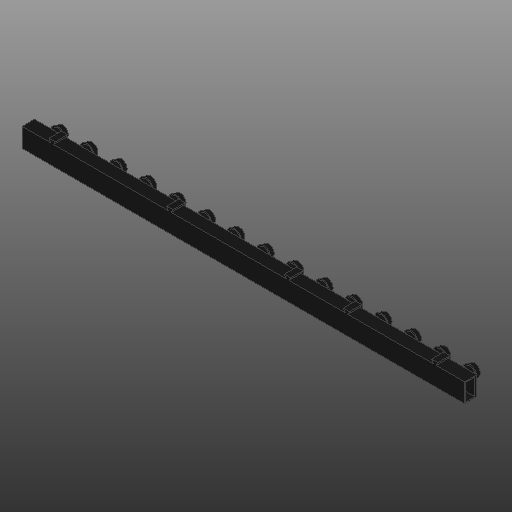
# Autodesk Inventor part: Manifold0
Saved by Autodesk Inventor 2020 (Build 240168000, 168)
## iProperties
Created: 2019-12-01
Part Number: Manifold0
Material: PLA Plastic (Black)
Document SubType Name: Modeling
Designer: Isaac Newcomb
Density: 1.06 g/cm^3
Appearance: 3D Printed - Black
Mass: 3.4119 g
Surface Area: 108.618 cm^2
Volume: 3.21878 cm^3
Project: Ice Keys
d33: 12.200 mm
d34: 2.533 mm
d35: 1.147 mm
d36: 1.300 mm
d37: 2.533 mm
d38: 1.147 mm
d39: 1.300 mm
d40: 2.533 mm
d41: 1.147 mm
d42: 1.300 mm
d43: 2.533 mm
d44: 1.147 mm
d45: 1.300 mm
d46: 2.533 mm
d47: 1.147 mm
d48: 1.300 mm
d53: 2.533 mm
d54: 1.147 mm
d55: 1.300 mm
d56: 2.533 mm
d57: 1.147 mm
d58: 1.300 mm
d61: 3.200 mm
d62: 1.600 mm
d63: 1.500 mm
d64: 3.200 mm
d65: 1.600 mm
d66: 1.500 mm
d67: 3.200 mm
d68: 1.600 mm
d69: 1.500 mm
d70: 3.200 mm
d71: 1.600 mm
d72: 1.500 mm
d73: 3.200 mm
d74: 1.600 mm
d75: 1.500 mm
d77: 0.400 mm
Author: Isaac Newcomb
Autodesk Inventor part; units mm, degrees
ref_plane "XZ Plane" through (0, 0, 0) normal (0, 1, 0) x (-1, 0, 0)
ref_plane "XY Plane" through (0, 0, 0) normal (0, 0, 1) x (1, 0, 0)
sketch "Box Sketch" plane through (0, 0, 0) normal (1, 0, 0) x (0, 1, 0)
  line L0 (0, 0) -> (7.7625, 0)
  line L1 (7.7625, 0) -> (7.7625, 5)
  line L2 (7.7625, 5) -> (0, 5)
  line L3 (0, 5) -> (0, 0)
  line L4 (0.4, 0.8) -> (7.3625, 0.8)
  line L5 (7.3625, 0.8) -> (7.3625, 4.6)
  line L6 (7.3625, 4.6) -> (0.4, 4.6)
  line L7 (0.4, 4.6) -> (0.4, 0.8)
  dimension "d0" = 0.8
  dimension "boxWallThick" = 0.4
  dimension "d2" = 0.4
  dimension "d3" = 0.4
  dimension "boxHeight" = 7.7625
  dimension "boxWidth" = 5
  constraints: 16 end point, 4 parallel, 2 horizontal, 2 perpendicular
  measures "d0" distance between parallel lines of L0 L4
  measures "boxWallThick" distance between parallel lines of L1 L5
  measures "d2" distance between parallel lines of L3 L7
  measures "d3" distance between parallel lines of L2 L6
  measures "boxHeight" distance of L0.start L0.end
  measures "boxWidth" distance of L2.end L0.start
extrude "Box" add sketch "Box Sketch" along normal blind 12.4
ref_plane "Fitting Plane" through (6.2, 0, 0) normal (1, 0, 0) x (0, 1, 0)
sketch "Fitting Sketch" plane through (6.2, 0, 0) normal (1, 0, 0) x (0, 1, 0)
  line L0 (3.8813, 0) -> (3.8813, -5.25) construction
  line L1 (5.4625, 0) -> (5.4625, -5.25)
  line L2 (5.4625, -5.25) -> (6.2625, -5.25)
  line L3 (6.2625, -5.25) -> (6.7625, -3.25)
  line L4 (6.7625, -3.25) -> (6.2625, -3.25)
  line L5 (6.2625, -3.25) -> (6.7625, -1.25)
  line L6 (6.7625, -1.25) -> (6.2625, -1.25)
  line L7 (6.2625, -1.25) -> (6.2625, 0)
  line L8 (6.2625, 0) -> (5.4625, 0)
  point P0 (0, 0)
  dimension "d10" = 2
  dimension "d11" = 0.5
  dimension "d12" = 1.25
  dimension "d13" = 0.8
  dimension "d14" = 2.3813
  dimension "d15" = 3.8813
  constraints: 18 end point, 5 point on line, 4 parallel, 3 perpendicular, 2 vertical
  measures "d10" distance between parallel lines of L6 L4
  measures "d11" distance of L3.end L4.end
  measures "d12" distance of L6.end L7.end
  measures "d13" distance of L1.end L2.end
  measures "d14" distance between parallel lines of L7 L0
  measures "d15" distance from line of point (0, 0) L0
revolve "Fitting" add sketch "Fitting Sketch" angle 360 about axis through (6.2, 3.8813, 0) along (0, 0, -1)
sketch "Fitting Entrance Sketch" plane through (6.2, 3.8813, 0) normal (0, 0, -1) x (-1, 0, 0)
  circle A0 centre (0, 0) radius 1.5813 projected
  point P0 (6.2, -3.8813)
extrude "Fitting Entrance" cut sketch "Fitting Entrance Sketch" against normal up to surface (0.8 mm away)
pattern_linear "Channel Repetition" count 15 spacing 12 along (1, 0, 0)
sketch "Tab Sketch" plane through (0, 0, 0) normal (0, 0, 1) x (1, 0, 0)
  line L0 (11.6267, 7.7625) -> (10.9333, 9.0625)
  line L1 (10.9333, 9.0625) -> (13.4667, 9.0625)
  line L2 (13.4667, 9.0625) -> (12.7733, 7.7625)
  line L3 (12.7733, 7.7625) -> (11.6267, 7.7625)
  line L4 (12.2, 7.7625) -> (12.2, 9.0625) construction
  line L5 (59.6267, 7.7625) -> (58.9333, 9.0625)
  line L6 (58.9333, 9.0625) -> (61.4667, 9.0625)
  line L7 (61.4667, 9.0625) -> (60.7733, 7.7625)
  line L8 (60.7733, 7.7625) -> (59.6267, 7.7625)
  line L9 (60.2, 7.7625) -> (60.2, 9.0625) construction
  line L10 (107.6267, 7.7625) -> (106.9333, 9.0625)
  line L11 (106.9333, 9.0625) -> (109.4667, 9.0625)
  line L12 (109.4667, 9.0625) -> (108.7733, 7.7625)
  line L13 (108.7733, 7.7625) -> (107.6267, 7.7625)
  line L14 (108.2, 7.7625) -> (108.2, 9.0625) construction
  line L15 (131.6267, 7.7625) -> (130.9333, 9.0625)
  line L16 (132.2, 7.7625) -> (132.2, 9.0625) construction
  line L17 (130.9333, 9.0625) -> (133.4667, 9.0625)
  line L18 (133.4667, 9.0625) -> (132.7733, 7.7625)
  line L19 (167.6267, 7.7625) -> (166.9333, 9.0625)
  line L20 (168.2, 7.7625) -> (168.2, 9.0625) construction
  line L21 (168.7733, 7.7625) -> (167.6267, 7.7625)
  line L22 (166.9333, 9.0625) -> (169.4667, 9.0625)
  line L23 (169.4667, 9.0625) -> (168.7733, 7.7625)
  line L24 (132.7733, 7.7625) -> (131.6267, 7.7625)
  line L25 (0, 7.7625) -> (0, 0) construction
  line L26 (11.4, 7.7625) -> (10.6, 9.2625)
  line L27 (10.6, 9.2625) -> (13.8, 9.2625)
  line L28 (13.8, 9.2625) -> (13, 7.7625)
  line L29 (13, 7.7625) -> (12.7733, 7.7625)
  line L30 (11.6267, 7.7625) -> (11.4, 7.7625)
  dimension "d33" = 12.2
  dimension "d34" = 2.5333
  dimension "d35" = 1.1467
  dimension "d36" = 1.3
  dimension "d37" = 2.5333
  dimension "d38" = 1.1467
  dimension "d39" = 1.3
  dimension "d40" = 2.5333
  dimension "d41" = 1.1467
  dimension "d42" = 1.3
  dimension "d43" = 2.5333
  dimension "d44" = 1.1467
  dimension "d45" = 1.3
  dimension "d46" = 2.5333
  dimension "d47" = 1.1467
  dimension "d48" = 1.3
  dimension "d49" = 48
  dimension "d50" = 48
  dimension "d51" = 24
  dimension "d52" = 36
  dimension "d79" = 7.7625
  dimension "d80" = 0.2
  dimension "d81" = 0.2
  dimension "d82" = 0.2
  dimension "d83" = 1.6
  dimension "d84" = 3.2
  dimension "d85" = 1.5
  constraints: 62 end point, 10 midpoint, 8 parallel, 6 horizontal, 5 collinear, 5 perpendicular, 1 point on line, 1 vertical
  measures "d33" distance from line of L25.start L4
  measures "d34" distance of L0.end L2.start
  measures "d35" distance of L2.end L3.end
  measures "d36" distance between parallel lines of L3 L1
  measures "d37" distance of L5.end L7.start
  measures "d38" distance of L7.end L8.end
  measures "d39" distance between parallel lines of L8 L6
  measures "d40" distance of L10.end L11.end
  measures "d41" distance of L12.end L10.start
  measures "d42" distance between parallel lines of L13 L11
  measures "d43" distance of L15.end L17.end
  measures "d44" distance of L24.start L15.start
  measures "d45" distance between parallel lines of L24 L17
  measures "d46" distance of L19.end L22.end
  measures "d47" distance of L21.start L19.start
  measures "d48" distance between parallel lines of L21 L22
  measures "d49" distance between parallel lines of L4 L9
  measures "d50" distance between parallel lines of L9 L14
  measures "d51" distance between parallel lines of L16 L14
  measures "d52" distance between parallel lines of L16 L20
  measures "d79" distance of L25.start L25.end
  measures "d80" distance between parallel lines of L2 L28
  measures "d81" distance between parallel lines of L27 L1
  measures "d82" distance between parallel lines of L26 L0
  measures "d83" distance of L28.end L26.start
  measures "d84" distance of L26.end L27.end
  measures "d85" distance between parallel lines of L3 L27
extrude "Tabs" add sketch "Tab Sketch" along normal blind 5 contours L0 L1 L2 L3 | L5 L6 L7 L8 | L10 L11 L12 L13 | L15 L17 L18 L24 | L19 L22 L23 L21
equation "\"d0\" = 2 * boxWallThick"
equation "\"boxWallThick\" = resoWallThick"
equation "\"d2\" = boxWallThick"
equation "\"d3\" = boxWallThick"
equation "\"boxHeight\" = 2 * fittingCtrOffset"
equation "\"boxWidth\" = manifoldWidth"
equation "\"d6\" = resoOuterDia"
equation "\"d10\" = fittingBarbLength"
equation "\"d11\" = fittingBarbHeight"
equation "\"d12\" = fittingNeckLength"
equation "\"d13\" = fittingWallThick"
equation "\"d14\" = fittingOuterRad"
equation "\"d15\" = 0.5 * boxHeight"
equation "\"d33\" = chanWidth + 0.5 * d77"
equation "\"d37\" = d34"
equation "\"d38\" = d35"
equation "\"d39\" = d36"
equation "\"d40\" = d34"
equation "\"d41\" = d35"
equation "\"d42\" = d36"
equation "\"d43\" = d34"
equation "\"d44\" = d35"
equation "\"d45\" = d36"
equation "\"d46\" = d34"
equation "\"d47\" = d35"
equation "\"d48\" = d36"
equation "\"d49\" = 4 * chanWidth"
equation "\"d50\" = 4 * chanWidth"
equation "\"d51\" = 2 * chanWidth"
equation "\"d52\" = 3 * chanWidth"
equation "\"d79\" = boxHeight"
equation "\"d80\" = tabTol"
equation "\"d81\" = tabTol"
equation "\"d82\" = tabTol"
equation "\"d83\" = slotBaseWidth"
equation "\"d84\" = slotTopWidth"
equation "\"d85\" = slotHeight"
equation "\"d31\" = boxWidth"
equation "\"d21\" = chanWidth"
equation "\"d8\" = 0.5 * resoOuterDia"
equation "\"d77\" = resoWallThick"
equation "\"tabTol\" = 0.2"
equation "\"resoWallThick\" = 0.4"
equation "\"fittingCtrOffset\" = 3.88125"
equation "\"manifoldWidth\" = 5"
equation "\"resoOuterDia\" = 12.4"
equation "\"fittingBarbLength\" = 2"
equation "\"fittingBarbHeight\" = 0.5"
equation "\"fittingNeckLength\" = 1.25"
equation "\"fittingWallThick\" = 0.8"
equation "\"fittingOuterRad\" = 2.38125"
equation "\"chanWidth\" = 12"
equation "\"slotBaseWidth\" = 1.6"
equation "\"slotTopWidth\" = 3.2"
equation "\"slotHeight\" = 1.5"
body "Solid1"
